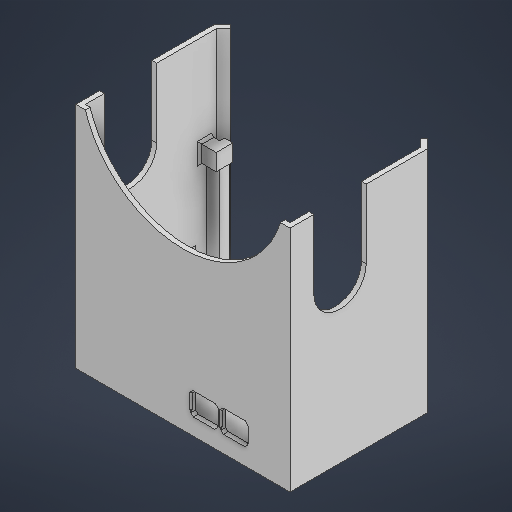
# Autodesk Inventor part: frame
Saved by Autodesk Inventor 2027.1 (Build 311270010, 270A)
## iProperties
Created: 2026-06-11
Part Number: frame
Material: Generic
Document SubType Name: Modeling
Designer: alexg
Density: 1 g/cm^3
Appearance: Default
Author: alexg
Autodesk Inventor part; units mm, degrees
ref_plane "YZ Plane" through (0, 0, 0) normal (1, 0, 0) x (0, 1, 0)
ref_plane "XZ Plane" through (0, 0, 0) normal (0, 1, 0) x (-1, 0, 0)
ref_plane "XY Plane" through (0, 0, 0) normal (0, 0, 1) x (1, 0, 0)
sketch "Sketch1" plane through (0, 0, 0) normal (0, 1, 0) x (-1, 0, 0)
  line L0 (-45, 30) -> (45, 30)
  line L1 (45, 30) -> (45, -30)
  line L2 (45, -30) -> (-45, -30)
  line L3 (-45, -30) -> (-45, 30)
  line L4 (-45, 30) -> (45, -30) construction
  line L5 (45, 30) -> (-45, -30) construction
  line L6 (43, 28) -> (-43, 28)
  line L7 (-43, 28) -> (-43, -28)
  line L8 (-43, -28) -> (43, -28)
  line L9 (43, -28) -> (43, 28)
  point P0 (0, 0)
  dimension "d0" = 90
  dimension "d1" = 60
  dimension "d2" = 86
  dimension "d3" = 56
  dimension "d4" = 2
  dimension "d5" = 2
  constraints: 20 end point, 4 parallel, 2 horizontal, 2 midpoint, 2 perpendicular
  measures "d0" distance of L1.end L2.end
  measures "d1" distance of L0.end L1.end
  measures "d2" distance of L8.end L7.end
  measures "d3" distance of L7.end L6.end
  measures "d4" distance between parallel lines of L2 L8
  measures "d5" distance between parallel lines of L3 L7
extrude "Extrusion1" add sketch "Sketch1" along normal blind 44
sketch "Sketch2" plane through (0, 0, 0) normal (0, -1, 0) x (1, 0, 0)
  line L0 (-45, 30) -> (45, 30) projected
  line L1 (-45, 30) -> (45, 30)
  line L2 (45, 30) -> (45, -30)
  line L3 (45, -30) -> (-45, -30)
  line L4 (-45, -30) -> (-45, 30)
  point P0 (0, 0)
  constraints: 8 end point, 2 parallel, 1 horizontal, 1 perpendicular
extrude "Extrusion2" add sketch "Sketch2" along normal blind 2
sketch "Sketch3" plane through (45, 44, 30) normal (1, 0, 0) x (0, 0, -1)
  line L0 (0, -46) -> (0, 0) projected
  line L1 (0, -22.505) -> (53, -22.505)
  line L2 (2, 0) -> (58, 0) projected
  line L3 (2, -44) -> (58, -44) projected
  line L4 (51, 0) -> (53, 0)
  line L5 (53, -44) -> (51, -44)
  line L6 (53, -44) -> (55, -44)
  line L7 (55, -44) -> (55, 0)
  line L8 (55, 0) -> (53, 0)
  line L9 (53, 0) -> (53, -44)
  point P0 (30, -44)
  dimension "d10" = 53
  dimension "d12" = 2
  constraints: 14 end point, 4 point on line, 3 horizontal, 3 parallel, 1 perpendicular
  measures "d10" distance of L1.start L1.end
  measures "d12" distance of L8.end L7.end
extrude "Extrusion3" add sketch "Sketch3" against normal blind 90
sketch "Sketch4" plane through (45, 44, -30) normal (0, 0, -1) x (-1, 0, 0)
  line L0 (2, 0) -> (88, 0) projected
  line L1 (88, -44) -> (2, -44) projected
  line L2 (2, 0) -> (88, 0)
  line L3 (88, 0) -> (88, -44)
  line L4 (88, -44) -> (2, -44)
  line L5 (2, -44) -> (2, 0)
  point P0 (45, -44)
  point P1 (2, -44)
  constraints: 8 end point, 2 parallel, 1 horizontal, 1 perpendicular
extrude "Extrusion4" cut sketch "Sketch4" against normal blind 2
sketch "Sketch5" plane through (43, 44, -25) normal (0, 0, -1) x (-1, 0, 0)
  line L0 (0, 0) -> (86, 0) projected
  line L1 (5.5, 0) -> (80.5, 0)
  line L2 (80.5, 0) -> (80.5, -44)
  line L3 (80.5, -44) -> (5.5, -44)
  line L4 (5.5, -44) -> (5.5, 0)
  line L5 (0, -44) -> (0, 0) projected
  point P0 (43, -44)
  dimension "d17" = 75
  dimension "d18" = 44
  dimension "d19" = 5.5
  constraints: 8 end point, 2 parallel, 1 horizontal, 1 perpendicular, 1 point on line
  measures "d17" distance of L2.end L3.end
  measures "d18" distance of L1.end L2.end
  measures "d19" distance between parallel lines of L5 L4
extrude "Extrusion5" cut sketch "Sketch5" against normal blind 2
sketch "Sketch6" plane through (-43, 0, -23) normal (0, 0, 1) x (1, 0, 0)
  line L0 (5.5, 0) -> (5.5, 44) projected
  line L1 (5.5, 44) -> (3.5, 44)
  line L2 (3.5, 44) -> (3.5, 0)
  line L3 (3.5, 0) -> (5.5, 0)
  line L4 (5.5, 0) -> (5.5, 44)
  line L5 (86, 44) -> (80.5, 44) projected
  line L6 (80.5, 44) -> (82.5, 44)
  line L7 (82.5, 44) -> (82.5, 0)
  line L8 (82.5, 0) -> (80.5, 0)
  line L9 (80.5, 0) -> (80.5, 44)
  point P0 (43, 0)
  dimension "d22" = 2
  dimension "d23" = 44
  dimension "d24" = 2
  dimension "d25" = 44
  constraints: 16 end point, 4 parallel, 2 horizontal, 2 perpendicular
  measures "d22" distance of L3.end L2.end
  measures "d23" distance of L2.end L1.end
  measures "d24" distance of L7.end L8.end
  measures "d25" distance of L6.end L7.end
extrude "Extrusion6" add sketch "Sketch6" against normal blind 4
sketch "Sketch8" plane through (45, -2, -30) normal (0, 0, -1) x (-1, 0, 0)
  line L0 (90, 46) -> (0, 46) projected
  line L1 (0, 46) -> (7.5, 46)
  line L2 (7.5, 46) -> (7.5, 0)
  line L3 (7.5, 0) -> (0, 0)
  line L4 (0, 0) -> (0, 46)
  line L5 (89.984, 46) -> (82.484, 46)
  line L6 (82.484, 46) -> (82.484, 0)
  line L7 (82.484, 0) -> (89.984, 0)
  line L8 (89.984, 0) -> (89.984, 46)
  point P0 (45, 2)
  point P1 (7.5, 46)
  dimension "d30" = 7.5
  dimension "d31" = 46
  dimension "d32" = 7.5
  dimension "d33" = 46
  constraints: 16 end point, 4 parallel, 2 horizontal, 2 perpendicular, 1 point on line
  measures "d30" distance of L2.end L3.end
  measures "d31" distance of L1.end L2.end
  measures "d32" distance of L7.end L6.end
  measures "d33" distance of L6.end L5.end
extrude "Extrusion7" cut sketch "Sketch8" against normal blind 1
sketch "Sketch9" plane through (-45, 44, -30) normal (-1, 0, 0) x (0, 0, 1)
  line L0 (0, -46) -> (0, 0) projected
  line L1 (1, 0) -> (1, -44) projected
  line L2 (0, -46) -> (1, -46)
  line L3 (1, -46) -> (1, 0)
  line L4 (1, 0) -> (0, 0)
  line L5 (0, 0) -> (0, -46)
  point P0 (30, -44)
  constraints: 8 end point, 2 parallel, 1 horizontal, 1 perpendicular
extrude "Extrusion8" cut sketch "Sketch9" against normal blind 1
sketch "Sketch10" plane through (0, 0, 0) normal (0, 1, 0) x (1, 0, 0)
  line L0 (-43, 25) -> (-43, 29) projected
  line L1 (-43, 27) -> (43, 27)
  line L2 (43, 29) -> (43, 25) projected
  line L3 (-43, 27) -> (-40, 30)
  line L4 (-43, 27) -> (-38.7574, 27) construction
  line L5 (-40, 30) -> (-41.4142, 31.4142)
  line L6 (-41.4142, 31.4142) -> (-45, 27.8284)
  line L7 (-45, -30) -> (-45, 29) projected
  line L8 (43, 27) -> (40, 30)
  line L9 (43, 27) -> (47.2426, 27) construction
  line L10 (40, 30) -> (41.4142, 31.4142)
  line L11 (40, 30) -> (42, 30) construction
  line L12 (41.4142, 31.4142) -> (45, 27.8284)
  line L13 (45, 27.8284) -> (43.2071, 26.7929)
  line L14 (-45, 29) -> (-37.484, 29) projected
  line L15 (-43.8284, 29) -> (-43, 29)
  line L16 (-43, 27) -> (-43, 29)
  line L17 (43, 29) -> (37.5, 29) projected
  line L18 (43, 27) -> (43, 29)
  line L19 (43, 29) -> (43.8284, 29)
  point P0 (0, 0)
  dimension "d38" = 45
  dimension "d39" = 2
  dimension "d40" = 90
  dimension "d41" = 90
  dimension "d42" = 135
  dimension "d43" = 2
  dimension "d44" = 45
  dimension "d45" = 90
  constraints: 30 end point, 5 perpendicular, 4 point on line, 3 equal length, 3 horizontal, 2 midpoint, 1 collinear
  measures "d38" angle of L4 L3
  measures "d39" distance of L3.end L5.end
  measures "d40" angle of L5 L3
  measures "d41" angle of L6 L5
  measures "d42" angle of L9 L8
  measures "d43" distance of L8.end L10.end
  measures "d44" angle of L11 L10
  measures "d45" angle of L10 L12
extrude "Extrusion9" add sketch "Sketch10" along normal blind 44 and the other way blind 2 contours L0 L14 L3 | L14 L6 L5 L3 | L2 L8 L17 | L17 L8 L10 L12 L19
sketch "Sketch11" plane through (0, 44, 0) normal (0, 1, 0) x (1, 0, 0)
  line L0 (37.5, 29) -> (45, 29) projected
  line L1 (43.8203, 29) -> (45, 29)
  line L2 (43.8284, 29) -> (45, 27.8284)
  line L3 (45, -30) -> (45, 29) projected
  line L4 (43.8284, 29) -> (45.4853, 29) construction
  line L5 (45, 27.8284) -> (45, 29)
  line L6 (-43.8284, 29) -> (-45, 29) projected
  line L7 (-43.8284, 29) -> (-45, 27.8284)
  line L8 (-45, 29) -> (-45, -30) projected
  line L9 (-43.8284, 29) -> (-42.1716, 29) construction
  line L10 (-45, 27.8284) -> (-45, 29)
  line L11 (-45, 29) -> (-43.8284, 29)
  point P0 (0, 0)
  dimension "d48" = 45
  dimension "d49" = 135
  constraints: 16 end point, 3 point on line, 2 collinear, 2 equal length, 2 horizontal, 1 perpendicular, 1 vertical
  measures "d48" angle of L2 L4
  measures "d49" angle of L7 L9
extrude "Extrusion10" cut sketch "Sketch11" against normal blind 48
sketch "Sketch12" plane through (-37.484, -2, -30) normal (-1, 0, 0) x (0, 0, 1)
  line L0 (1, 0) -> (1, 2) projected
  line L1 (0, 0) -> (0, 2) projected
  line L2 (1, 2) -> (0, 2)
  line L3 (0, 2) -> (0, 0)
  line L4 (0, 0) -> (1, 0)
  line L5 (1, 0) -> (1, 2)
  point P0 (30, 2)
  constraints: 8 end point, 2 parallel, 1 horizontal, 1 perpendicular
extrude "Extrusion11" add sketch "Sketch12" along normal blind 4.5 and the other way blind 79
sketch "Sketch13" plane through (0, 0, 0) normal (0, 1, 0) x (1, 0, 0)
  circle A0 centre (0, 26.5) radius 2
  line L0 (-40, 30) -> (40, 30) projected
  point P0 (0, 0)
  point P1 (0, 30)
  dimension "d58" = 4
  dimension "d59" = 3.5
  constraints: 1 centre point, 1 midpoint
  measures "d58" diameter of A0
  measures "d59" distance of point (0, 30) A0.centre
extrude "Extrusion12" cut sketch "Sketch13" against normal blind 4.5
sketch "Sketch14" plane through (0, 44, 0) normal (0, 1, 0) x (1, 0, 0)
  line L0 (45, -30) -> (-45, -30) projected
  line L1 (45, -30) -> (-45, -30)
  line L2 (-45, -30) -> (-45, 27.8284)
  line L3 (-41.4142, 31.4142) -> (-40, 30) projected
  line L4 (-45, 27.8284) -> (-41.4142, 31.4142)
  line L5 (-41.4142, 31.4142) -> (-40, 30)
  line L6 (-43, 27) -> (-40, 30)
  line L7 (43, -28) -> (-43, -28) projected
  line L8 (-43, 27) -> (-43, -28)
  line L9 (43, -28) -> (43, 27)
  line L10 (45, 27.8284) -> (45, -30) projected
  line L11 (40, 30) -> (43, 27) projected
  line L12 (43, 27) -> (40, 30)
  line L13 (40, 30) -> (41.4142, 31.4142) projected
  line L14 (40, 30) -> (41.4142, 31.4142)
  line L15 (41.4142, 31.4142) -> (45, 27.8284)
  point P0 (0, 0)
  constraints: 20 end point, 5 perpendicular, 3 collinear, 1 parallel, 1 vertical
extrude "Extrusion13" add sketch "Sketch14" along normal blind 50
sketch "Sketch15" plane through (43, 0, 28) normal (0, 0, -1) x (-1, 0, 0)
  circle A0 centre (43, 107) radius 43
  line L0 (0, 94) -> (86, 94) projected
  point P0 (43, 0)
  point P1 (83.9878, 94)
  point P2 (2.0122, 94)
  dimension "d64" = 86
  dimension "d65" = 13
  constraints: 1 centre point
  measures "d64" diameter of A0
  measures "d65" distance from line of L0 A0.centre
extrude "Extrusion14" cut sketch "Sketch15" against normal blind 16 contours L0 A0 picked at (43, 84)
sketch "Sketch16" plane through (-43, 0, 28) normal (1, 0, 0) x (0, 0, -1)
  circle A0 centre (19, 65) radius 11
  line L0 (0, 94) -> (55, 94) projected
  line L1 (0, 94) -> (0, 64) projected
  line L2 (8, 65) -> (8, 94)
  line L3 (30, 65) -> (30, 94)
  point P0 (28, 0)
  dimension "d68" = 22
  dimension "d69" = 29
  dimension "d70" = 19
  constraints: 4 end point, 2 perpendicular, 2 point on circle, 2 point on line, 2 tangent, 1 centre point
  measures "d68" diameter of A0
  measures "d69" distance from line of L0 A0.centre
  measures "d70" distance from line of L1 A0.centre
sketch "Sketch17" plane through (43, 0, -23) normal (-1, 0, 0) x (0, 0, 1)
  circle A0 centre (32, 65) radius 11
  line L0 (-4, 94) -> (51, 94) projected
  line L1 (51, 0) -> (51, 94) projected
  line L2 (43, 65) -> (43, 94)
  line L3 (43, 65) -> (72, 65) construction
  line L4 (21, 65) -> (21, 94)
  line L5 (21, 65) -> (50, 65) construction
  line L6 (21, 94) -> (43, 94)
  point P0 (23, 0)
  dimension "d71" = 22
  dimension "d72" = 29
  dimension "d73" = 19
  dimension "d74" = 90
  dimension "d75" = 90
  constraints: 10 end point, 2 horizontal, 2 perpendicular, 2 point on circle, 2 point on line, 1 centre point, 1 collinear
  measures "d71" diameter of A0
  measures "d72" distance from line of L0 A0.centre
  measures "d73" distance from line of L1 A0.centre
  measures "d74" angle of L3 L2
  measures "d75" angle of L5 L4
extrude "Extrusion15" cut sketch "Sketch17" against normal blind 16
extrude "Extrusion16" cut sketch "Sketch16" against normal blind 16
sketch "Sketch18" plane through (-43, 0, 28) normal (1, 0, 0) x (0, 0, -1)
  point P0 (28, 0)
chamfer "Chamfer1" distance 2 angle 45 3 edges at (0, 0, 28) (43, 0, 2.5) (-43, 0, 2.5)
sketch "Sketch19" plane through (0, 0, 0) normal (0, 1, 0) x (1, 0, 0)
  line L0 (32.5, -26) -> (-32.5, -26)
  line L1 (-32.5, -26) -> (-32.5, 4)
  line L2 (-32.5, 4) -> (32.5, 4)
  line L3 (32.5, 4) -> (32.5, -26)
  line L4 (41, 23) -> (41, -26) projected
  line L5 (41, -26) -> (-41, -26) projected
  circle A0 centre (29, 0.5) radius 1
  circle A1 centre (-29, 0.5) radius 1
  circle A2 centre (-29, -22.5) radius 1
  circle A3 centre (29, -22.5) radius 1
  circle A4 centre (29, 0.5) radius 2.5
  circle A5 centre (-29, 0.5) radius 2.5
  circle A6 centre (-29, -22.5) radius 2.5
  circle A7 centre (29, -22.5) radius 2.5
  point P0 (0, 0)
  dimension "d83" = 65
  dimension "d84" = 30
  dimension "d85" = 8.5
  dimension "d86" = 0
  dimension "d87" = 2
  dimension "d88" = 2
  dimension "d89" = 2
  dimension "d90" = 2
  dimension "d91" = 3.5
  dimension "d92" = 3.5
  dimension "d93" = 3.5
  dimension "d94" = 3.5
  dimension "d95" = 3.5
  dimension "d96" = 3.5
  dimension "d97" = 3.5
  dimension "d98" = 3.5
  dimension "d99" = 5
  dimension "d100" = 5
  dimension "d101" = 5
  dimension "d102" = 5
  constraints: 8 centre point, 8 end point, 4 coincident, 2 parallel, 1 horizontal, 1 perpendicular
  measures "d83" distance of L1.end L2.end
  measures "d84" distance of L0.end L1.end
  measures "d85" distance between parallel lines of L4 L3
  measures "d86" distance between parallel lines of L5 L0
  measures "d87" diameter of A0
  measures "d88" diameter of A1
  measures "d89" diameter of A2
  measures "d90" diameter of A3
  measures "d91" distance from line of L2 A0.centre
  measures "d92" distance from line of L3 A0.centre
  measures "d93" distance from line of L3 A3.centre
  measures "d94" distance from line of L5 A3.centre
  measures "d95" distance from line of L5 A2.centre
  measures "d96" distance from line of L1 A2.centre
  measures "d97" distance from line of L1 A1.centre
  measures "d98" distance from line of L2 A1.centre
  measures "d99" diameter of A4
  measures "d100" diameter of A5
  measures "d101" diameter of A6
  measures "d102" diameter of A7
extrude "Extrusion17" add sketch "Sketch19" along normal blind 5 contours A4 | A5 | A6 | A7
sketch "Sketch20" plane through (0, 107, 28) normal (0, 0, -1) x (-1, 0, 0)
  line L0 (-26.5, -102) -> (-31.5, -102) projected
  line L1 (39.5, -63) -> (39.5, -107) projected
  line L2 (-31.5, -101) -> (39.5, -101) construction
  line L3 (-39.5, -107) -> (-39.5, -63) projected
  line L4 (28, -102) -> (30, -102) projected
  line L5 (29, -102) -> (30, -102) construction
  line L6 (29, -101) -> (79.5, -101) construction
  line L7 (-3.4, -97) -> (-3.4, -101)
  line L8 (-3.4, -101) -> (-14.4, -101)
  line L9 (-14.4, -101) -> (-14.4, -97)
  line L10 (-14.4, -97) -> (-3.4, -101) construction
  line L11 (-3.4, -97) -> (-14.4, -101) construction
  line L12 (-16, -97) -> (-16, -101)
  line L13 (-16, -101) -> (-27, -101)
  line L14 (-27, -101) -> (-27, -97)
  line L15 (-27, -97) -> (-16, -101) construction
  line L16 (-16, -97) -> (-27, -101) construction
  line L17 (-16, -97) -> (-16, -93)
  line L18 (-16, -93) -> (-27, -93)
  line L19 (-27, -93) -> (-27, -97)
  line L20 (-3.4, -97) -> (-3.4, -93)
  line L21 (-3.4, -93) -> (-14.4, -93)
  line L22 (-14.4, -93) -> (-14.4, -97)
  point P0 (0, -107)
  point P1 (-8.9, -99)
  point P2 (-21.5, -99)
  point P3 (-16, -97)
  dimension "d123" = 4
  dimension "d125" = 4
  dimension "d126" = 5.5
  dimension "d127" = 5.5
  dimension "d128" = 11
  dimension "d129" = 4
  dimension "d130" = 11
  dimension "d131" = 4
  constraints: 38 end point, 5 midpoint, 4 parallel, 3 horizontal
  measures "d123" distance of L7.start L7.end
  measures "d125" distance of L12.start L12.end
  measures "d126" distance from line of L12 point (-21.5, -99)
  measures "d127" distance from line of L9 point (-8.9, -99)
  measures "d128" distance of L18.end L17.end
  measures "d129" distance of L17.end L17.start
  measures "d130" distance of L21.end L20.end
  measures "d131" distance of L20.end L20.start
extrude "Extrusion18" cut sketch "Sketch20" against normal blind 2
chamfer "Chamfer2" distance 1 angle 45 8 edges at (27, 6, 29) (27, 14, 29) (16, 14, 29) (16, 6, 29) (14.4, 6, 29) (14.4, 14, 29) (3.4, 14, 29) (3.4, 6, 29)
chamfer "Chamfer3" distance 0.5 angle 45 16 edges at (16.5, 13.5, 30) (21.5, 14, 30) (26.5, 13.5, 30) (27, 10, 30) (26.5, 6.5, 30) (21.5, 6, 30) (16.5, 6.5, 30) (16, 10, 30) (14.4, 10, 30) (13.9, 6.5, 30) (13.9, 13.5, 30) (8.9, 14, 30) (8.9, 6, 30) (3.4, 10, 30) (3.9, 13.5, 30) (3.9, 6.5, 30)
sketch "Sketch22" plane through (43, 0, -25) normal (-1, 0, 0) x (0, 0, 1)
  line L0 (27, 0) -> (27, 5) projected
  line L1 (45, 0) -> (45, 5) projected
  line L2 (27, 2.0078) -> (36, 2.0078) construction
  line L3 (36, 2.0078) -> (51, 2.0078) construction
  line L4 (2, 2) -> (51, 2) projected
  line L5 (45.0001, 2) -> (40.0001, 2)
  line L6 (45.0001, 2) -> (50.0001, 2) construction
  line L7 (40.0001, 17) -> (9.0001, 17)
  line L8 (7.5001, 15.5) -> (10.5001, 15.5)
  line L9 (10.5001, 15.5) -> (10.5001, 18.5)
  line L10 (10.5001, 18.5) -> (7.5001, 18.5)
  line L11 (7.5001, 18.5) -> (7.5001, 15.5)
  line L12 (7.5001, 15.5) -> (10.5001, 18.5) construction
  line L13 (10.5001, 15.5) -> (7.5001, 18.5) construction
  line L14 (41.5001, 15.5) -> (38.5001, 15.5)
  line L15 (38.5001, 15.5) -> (38.5001, 18.5)
  line L16 (38.5001, 18.5) -> (41.5001, 18.5)
  line L17 (41.5001, 18.5) -> (41.5001, 15.5)
  line L18 (41.5001, 15.5) -> (38.5001, 18.5) construction
  line L19 (38.5001, 15.5) -> (41.5001, 18.5) construction
  point P0 (25, 0)
  dimension "d150" = 15
  dimension "d152" = 31
  dimension "d154" = 3
  dimension "d155" = 3
  dimension "d156" = 3
  dimension "d157" = 3
  constraints: 34 end point, 5 horizontal, 4 midpoint, 4 parallel, 2 collinear, 2 perpendicular, 2 point on line
  measures "d150" distance of L5.end L7.start
  measures "d152" distance of L7.start L7.end
  measures "d154" distance of L10.end L9.end
  measures "d155" distance of L9.end L8.end
  measures "d156" distance of L15.end L16.end
  measures "d157" distance of L14.end L15.end
extrude "Extrusion20" add sketch "Sketch22" along normal blind 87
sketch "Sketch23" plane through (0, 107, 28) normal (0, 0, -1) x (-1, 0, 0)
  line L0 (-27, -94) -> (-27, -100) projected
  line L1 (-27, -100) -> (-16, -100)
  line L2 (-16, -100) -> (-16, -102)
  line L3 (-16, -102) -> (-27, -102)
  line L4 (-27, -102) -> (-27, -100)
  line L5 (-14.4, -100) -> (-13.4, -101) projected
  line L6 (-14.4, -100) -> (-3.4, -100)
  line L7 (-3.4, -100) -> (-3.4, -102)
  line L8 (-3.4, -102) -> (-14.4, -102)
  line L9 (-14.4, -102) -> (-14.4, -100)
  point P0 (0, -107)
  dimension "d160" = 11
  dimension "d161" = 2
  dimension "d162" = 11
  dimension "d163" = 2
  constraints: 16 end point, 4 parallel, 2 horizontal, 2 perpendicular
  measures "d160" distance of L2.end L3.end
  measures "d161" distance of L1.end L2.end
  measures "d162" distance of L7.end L8.end
  measures "d163" distance of L6.end L7.end
extrude "Extrusion21" cut sketch "Sketch23" against normal blind 87
chamfer "Chamfer4" distance 1 angle 45 4 edges at (14.4, 5, 29) (27, 5, 29) (3.4, 5, 29) (16, 5, 29)
sketch "Sketch24" plane through (43, 18.5, -14.4999) normal (0, 1, 0) x (1, 0, 0)
  line L0 (-2, -40.4999) -> (-84, -40.4999) projected
  circle A0 centre (-15.75, -29.5) radius 1
  line L1 (0, -28) -> (-86, -28) projected
  circle A1 centre (-70.25, -29.5) radius 1
  circle A2 centre (-15.75, 1.5) radius 1
  line L2 (0, 3) -> (-86, 3) projected
  circle A3 centre (-70.25, 1.5) radius 1
  line L3 (0, 0) -> (-86, 0) projected
  circle A4 centre (-15.75, -29.5) radius 3
  circle A5 centre (-70.25, -29.5) radius 3
  circle A6 centre (-70.25, 1.5) radius 3
  circle A7 centre (-15.75, 1.5) radius 3
  point P0 (-43, -14.4999)
  point P1 (-43, -29.4179)
  dimension "d172" = 2
  dimension "d174" = 1.5
  dimension "d175" = 2
  dimension "d176" = 1.5
  dimension "d178" = 2
  dimension "d180" = 1.5
  dimension "d181" = 2
  dimension "d182" = 1.5
  dimension "d184" = 6
  dimension "d185" = 6
  dimension "d186" = 6
  dimension "d187" = 6
  constraints: 8 centre point, 4 coincident
  measures "d172" diameter of A0
  measures "d174" distance from line of L1 A0.centre
  measures "d175" diameter of A1
  measures "d176" distance from line of L1 A1.centre
  measures "d178" diameter of A2
  measures "d180" distance from line of L2 A2.centre
  measures "d181" diameter of A3
  measures "d182" distance from line of L3 A3.centre
  measures "d184" diameter of A4
  measures "d185" diameter of A5
  measures "d186" diameter of A6
  measures "d187" diameter of A7
extrude "Extrusion22" add sketch "Sketch24" along normal blind 1 and the other way blind 4 contours A4 L1 | L1 A4 | A5 L1 | L1 A5 | A7 L3 L2 | L2 A7 | A6 L3 L2 | L2 A6 | L3 A7 | A6 L3
chamfer "Chamfer5" distance 1 angle 45 8 edges at (43, 18.5, 15.0001) (43, 17, 13.5001) (43, 18.5, -15.9999) (43, 17, -17.4999) (43, 15.5, 15.0001) (43, 15.5, -15.9999) (43, 17, -14.4999) (43, 17, 16.5001)
chamfer "Chamfer6" distance 1 angle 45 6 edges at (-43, 18.5, -15.9999) (-43, 17, -17.4999) (-43, 18.5, 15.0001) (-43, 17, 13.5001) (-43, 17, 16.5001) (-43, 17, -14.4999)
chamfer "Chamfer7" distance 1 angle 45 6 edges at (-43, 15.5, -17.9999) (-43, 15.5, -15.9999) (-43, 15.5, -13.9999) (-43, 15.5, 13.0001) (-43, 15.5, 15.0001) (-43, 15.5, 17.0001)
sketch "Sketch27" plane through (43, 0, -25) normal (-1, 0, 0) x (0, 0, 1)
  line L0 (37.5001, 19.5) -> (38.5001, 18.5) projected
  line L1 (37.5001, 49) -> (53, 48.5)
  line L2 (53, 2) -> (53, 94) projected
  line L3 (37.5001, 49) -> (-2, 49)
  line L4 (-2, 2) -> (-2, 94) projected
  line L5 (-2, 49) -> (5, 49)
  line L6 (5, 49) -> (5, 56)
  line L7 (5, 56) -> (-2, 56)
  line L8 (-2, 56) -> (-2, 49)
  line L9 (53, 48.5) -> (46, 48.5)
  line L10 (46, 48.5) -> (46, 55.5)
  line L11 (46, 55.5) -> (53, 55.5)
  line L12 (53, 55.5) -> (53, 48.5)
  point P0 (25, 0)
  point P1 (46, 48.7258)
  point P2 (5, 49)
  dimension "d207" = 7
  dimension "d208" = 7
  dimension "d209" = 7
  dimension "d210" = 7
  constraints: 20 end point, 4 parallel, 2 horizontal, 2 perpendicular, 2 point on line
  measures "d207" distance of L7.end L6.end
  measures "d208" distance of L6.end L5.end
  measures "d209" distance of L10.end L11.end
  measures "d210" distance of L9.end L10.end
extrude "Extrusion24" add sketch "Sketch27" along normal blind 7 contours L10 L11 L2 L1 | L3 L4 L7 L6
sketch "Sketch31" plane through (-43, 0, -25) normal (1, 0, 0) x (0, 0, -1)
  line L0 (0, 44) -> (-2, 44) projected
  line L1 (0, 44) -> (0, 49)
  line L2 (0, 49) -> (-64.6898, 49)
  line L3 (-64.6898, 49) -> (3.817, 49)
  line L4 (2, 0) -> (2, 94) projected
  line L5 (2, 49) -> (-5, 49)
  line L6 (-5, 49) -> (-5, 56)
  line L7 (-5, 56) -> (2, 56)
  line L8 (2, 56) -> (2, 49)
  line L9 (-53, 2) -> (-53, 94) projected
  line L10 (-53, 49) -> (-46, 49)
  line L11 (-46, 49) -> (-46, 56)
  line L12 (-46, 56) -> (-53, 56)
  line L13 (-53, 56) -> (-53, 49)
  point P0 (-25, 0)
  point P1 (2, 56)
  point P2 (-53, 56)
  point P3 (-53, 49)
  point P4 (-46, 49)
  dimension "d217" = 5
  dimension "d218" = 90
  dimension "d219" = 7
  dimension "d220" = 7
  dimension "d221" = 7
  dimension "d222" = 7
  constraints: 22 end point, 5 point on line, 4 parallel, 2 horizontal, 2 perpendicular, 1 vertical
  measures "d217" distance of L0.start L1.end
  measures "d218" angle of L2 L1
  measures "d219" distance of L6.end L7.end
  measures "d220" distance of L5.end L6.end
  measures "d221" distance of L12.end L11.end
  measures "d222" distance of L11.end L10.end
extrude "Extrusion26" add sketch "Sketch31" along normal blind 7
chamfer "Chamfer8" distance 1 angle 45 9 edges at (-39.5, 56, 28) (-43, 56, 24.5) (-43, 56, -23.5) (-43, 52.5, 21) (-36, 52.5, 28) (-39.5, 49, 28) (-43, 49, 24.5) (-43, 49, -23.5) (-43, 52.5, -20)
chamfer "Chamfer9" distance 1 angle 45 4 edges at (39.5, 55.5, 28) (43, 55.5, 24.5) (43, 52.1129, 21) (36, 52, 28)
chamfer "Chamfer10" distance 1 angle 45 4 edges at (35.5, 48.5, 28) (39.5, 48.5, 28) (43, 48.7419, 20.5) (43, 48.6129, 24.5)
chamfer "Chamfer11" distance 1 angle 45 2 edges at (43, 49, -23.5) (43, 56, -23.5)
chamfer "Chamfer12" distance 1 angle 45 3 edges at (43, 48.5, -20) (43, 52.5, -20) (43, 56.5, -20)
sketch "Sketch32" plane through (0, 44, 0) normal (0, 1, 0) x (1, 0, 0)
  line L0 (43, 23) -> (43, 25) projected
  line L1 (43, 25) -> (39.5, 25)
  line L2 (39.5, 25) -> (39.5, 27) projected
  line L3 (39.5, 25) -> (39.5, 27)
  line L4 (39.5, 27) -> (43, 27)
  line L5 (43, 27) -> (43, 25)
  line L6 (-39.5, 25) -> (-43, 25) projected
  line L7 (-43, 25) -> (-39.5, 25)
  line L8 (-39.5, 27) -> (-37.5, 27) projected
  line L9 (-39.5, 25) -> (-39.5, 27)
  line L10 (-39.5, 27) -> (-43, 27)
  line L11 (-43, 27) -> (-43, 25)
  point P0 (0, 0)
  dimension "d240" = 90
  dimension "d241" = 90
  constraints: 16 end point, 5 perpendicular, 1 collinear, 1 horizontal
  measures "d240" angle of L3 L4
  measures "d241" angle of L10 L9
extrude "Extrusion27" cut sketch "Sketch32" along normal blind 50
sketch "Sketch33" plane through (0, 44, 0) normal (0, 1, 0) x (1, 0, 0)
  line L0 (-43, 25) -> (-43, 23) projected
  line L1 (-43, 23) -> (-43, 25)
  line L2 (-37.5, 23) -> (-43, 23) projected
  line L3 (-39.5, 25) -> (-39.5, 27) projected
  line L4 (-37.5, 23) -> (-39.5, 23)
  line L5 (-39.5, 23) -> (-39.5, 27)
  line L6 (-39.5, 27) -> (-37.5, 27)
  line L7 (-37.5, 27) -> (-37.5, 23)
  line L8 (-39.5, 23) -> (-43, 23)
  line L9 (-43, 23) -> (-43, 25)
  line L10 (-43, 25) -> (-39.5, 25)
  line L11 (-39.5, 25) -> (-39.5, 23)
  line L12 (43, 23) -> (37.5, 23) projected
  line L13 (43, 23) -> (39.5, 23)
  line L14 (39.5, 23) -> (39.5, 25)
  line L15 (39.5, 25) -> (43, 25)
  line L16 (43, 25) -> (43, 23)
  line L17 (39.5, 25) -> (39.5, 27) projected
  line L18 (39.5, 27) -> (37.5, 27)
  line L19 (37.5, 27) -> (37.5, 23)
  line L20 (37.5, 23) -> (39.5, 23)
  line L21 (39.5, 23) -> (39.5, 27)
  point P0 (0, 0)
  constraints: 34 end point, 8 parallel, 4 horizontal, 4 perpendicular, 1 point on line, 1 vertical
extrude "Extrusion28" add sketch "Sketch33" along normal blind 5 contours L10 L5 L2 L0 | L3 L6 L7 L2 L5
sketch "Sketch34" plane through (0, 44, 0) normal (0, 1, 0) x (1, 0, 0)
  line L0 (43, 23) -> (37.5, 23) projected
  line L1 (43, 23) -> (39.5, 23)
  line L2 (39.5, 23) -> (39.5, 25)
  line L3 (39.5, 25) -> (43, 25)
  line L4 (43, 25) -> (43, 23)
  point P0 (0, 0)
  dimension "d246" = 3.5
  dimension "d247" = 2
  constraints: 8 end point, 2 parallel, 1 horizontal, 1 perpendicular
  measures "d246" distance of L2.end L3.end
  measures "d247" distance of L1.end L2.end
extrude "Extrusion29" add sketch "Sketch34" along normal blind 5
sketch "Sketch35" plane through (0, 44, 0) normal (0, 1, 0) x (1, 0, 0)
  line L0 (39.5, 23) -> (39.5, 25) projected
  line L1 (37.5, 23) -> (37.5, 27) projected
  line L2 (39.5, 23) -> (37.5, 23)
  line L3 (37.5, 23) -> (37.5, 27)
  line L4 (37.5, 27) -> (39.5, 27)
  line L5 (39.5, 27) -> (39.5, 23)
  point P0 (0, 0)
  constraints: 8 end point, 2 parallel, 1 horizontal, 1 perpendicular
extrude "Extrusion30" add sketch "Sketch35" along normal blind 5
chamfer "Chamfer13" distance 1 angle 45 1 edges at (37.5, 49, -25)
chamfer "Chamfer14" distance 1 angle 45 1 edges at (-37.5, 49, -25)
chamfer "Chamfer15" distance 1 angle 45 2 edges at (-37, 49, -23) (-39.75, 49, -23)
chamfer "Chamfer16" distance 1 angle 45 3 edges at (40.75, 49, -23) (37, 49, -23) (38.5, 49, -23)
body "Solid1"
